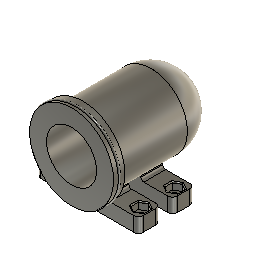
POP_MainBody_Extended_Feet (Autodesk Fusion 360 design; units mm, degrees)
Autodesk Fusion 360 part; units mm, degrees
sketch "Sketch1" plane through (0, 0, 0) normal (0, 1, 0) x (1, 0, 0)
  circle A0 centre (0, 0) radius 22
  circle A1 centre (0, 0) radius 32
  dimension "d1" = 44
  dimension "d2" = 10
  constraint coincident A0.centre A1.centre
  measures "d1" diameter of A0
extrude "Extrude1" add sketch "Sketch1" along normal blind 70 makes body 1
sketch "Sketch2" plane through (0, 0, 0) normal (0, 0, 1) x (1, 0, 0)
  line L0 (0, 0) -> (0, 97.6409) construction
  line L1 (0, 69.4626) -> (31, 69.4626)
  arc A0 (0, 91.4626) -> (-22, 69.4626) centre (0, 69.4626) ccw
  arc A1 (0, 101.4626) -> (-32, 69.4626) centre (0, 69.4626) ccw
  line L2 (0, 69.4626) -> (-32, 69.4626) construction
  line L3 (31, 69.4626) -> (21, 69.4626)
  line L4 (-22, 69.4626) -> (-32, 69.4626)
  line L5 (0, 91.4626) -> (0, 101.4626)
  dimension "d7" = 32
  dimension "d8" = 22
  constraint coincident L0.start origin
  constraint vertical L0
  constraint coincident L1.start L0
  constraint coincident L1.start A0.centre
  constraint perpendicular L0 L1
  constraint concentric A0 A1
  constraint coincident L1 L3.end
  constraint perpendicular L0 L2
  constraint coincident L2 A0.end
  measures "d7" radius of A1
  measures "d8" radius of A0
revolve "Revolve1" add sketch "Sketch2" angle 360 about axis through (0, 0, 0) along (0, 1, 0) bodies 1
sketch "Sketch3" plane through (0, 0, 0) normal (0, -1, 0) x (1, 0, 0)
  circle A0 centre (0, 0) radius 22
  circle A1 centre (0, 0) radius 32
  circle A2 centre (0, 0) radius 25.146 construction
  circle A3 centre (0, 0) radius 28.702 construction
  dimension "d10" = 50.292
  dimension "d11" = 57.404
  constraint coincident A0.centre A1.centre
  measures "d10" diameter of A2
  measures "d11" diameter of A3
ref_plane "WorkPlane1" through (0, 37.5401, -32) normal (0, 0, -1) x (1, 0, 0)
sketch "Sketch4" plane through (0, 37.5401, -32) normal (0, 0, -1) x (1, 0, 0)
  line L0 (45, 23.5401) -> (-45, 23.5401)
  line L1 (-45, 23.5401) -> (-45, 4.2401)
  line L2 (-45, 4.2401) -> (45, 4.2401)
  line L3 (45, 4.2401) -> (45, 23.5401)
  line L4 (45, 23.5401) -> (-45, 4.2401) construction
  line L5 (-45, 23.5401) -> (45, 4.2401) construction
  line L6 (0, 0) -> (0, 37.5401) construction
  line L7 (0, 0) -> (0, -48.773) construction
  circle A0 centre (-37.35, 13.8901) radius 3.302
  circle A1 centre (37.35, 13.8901) radius 3.302
  point P0 (0, 13.8901)
  point P1 (0, 37.5401)
  dimension "d13" = 90
  dimension "d14" = 19.3
  dimension "d15" = 14
  dimension "d16" = 6.604
  dimension "d17" = 7.65
  dimension "d18" = 6.604
  dimension "d19" = 7.65
  dimension "d20" = 9.65
  dimension "d21" = 9.65
  constraint horizontal L0
  constraint perpendicular L0 L1
  constraint parallel L0 L2
  constraint parallel L1 L3
  constraint coincident L4 P0
  constraint coincident L5 P0
  constraint midpoint L5 P0
  constraint coincident L6.start L7.start
  constraint perpendicular L0 L6
  constraint coincident P0 L6
  constraint parallel L6 L7
  constraint coincident P1 L6.end
  measures "d13" distance of L0.start L0.end
  measures "d14" distance of L0.end L1.end
  measures "d15" distance of L0 P1
  measures "d16" diameter of A0
  measures "d17" distance of L1 A0.centre
  measures "d18" diameter of A1
  measures "d19" distance of L3 A1.centre
  measures "d20" distance of L0 A0.centre
  measures "d21" distance of L0 A1.centre
extrude "Extrude2" add sketch "Sketch4" against normal blind 12.7 from surface at 12.7 separate body makes body 2
sketch "Sketch11" plane through (0, 0, -32) normal (0, 0, 1) x (-1, 0, 0)
  circle A0 centre (-37.35, -23.65) radius 3.302
  circle A1 centre (37.35, -23.65) radius 3.302
  line L0 (-45, -14) -> (-45, -33.3)
  line L1 (-45, -33.3) -> (45, -33.3)
  line L2 (45, -33.3) -> (45, -14)
  line L3 (45, -14) -> (-45, -14)
  line L4 (-42.938, -20.4238) -> (-42.938, -26.8762)
  line L5 (-42.938, -26.8762) -> (-37.35, -30.1025)
  line L6 (-37.35, -30.1025) -> (-31.762, -26.8762)
  line L7 (-31.762, -26.8762) -> (-31.762, -20.4238)
  line L8 (-31.762, -20.4238) -> (-37.35, -17.1975)
  line L9 (-37.35, -17.1975) -> (-42.938, -20.4238)
  line L10 (0, -33.3) -> (0, -14) construction
  line L11 (42.938, -26.8762) -> (37.35, -30.1025)
  line L12 (42.938, -20.4238) -> (42.938, -26.8762)
  line L13 (37.35, -17.1975) -> (42.938, -20.4238)
  line L14 (31.762, -20.4238) -> (37.35, -17.1975)
  line L15 (31.762, -26.8762) -> (31.762, -20.4238)
  line L16 (37.35, -30.1025) -> (31.762, -26.8762)
  point P0 (-37.35, -23.65)
  dimension "d77" = 11.176
  constraint coincident P0 A0.centre
  constraint vertical L4
  constraint midpoint L1 L10.start
  constraint midpoint L3 L10.end
  constraint symmetric L4.start L10 L12.start
  constraint symmetric L4.end L10 L11.start
  constraint symmetric L5.end L10 L11.end
  constraint symmetric L6.end L10 L15.start
  constraint symmetric L7.end L10 L14.start
  constraint symmetric L8.end L10 L13.start
  measures "d77" distance of L4 L7
extrude "Extrude9" cut sketch "Sketch11" against normal blind 6.35 contours L4 L5 L6 L7 L8 L9 | L11 L12 L13 L14 L15 L16 bodies 2
fillet "Fillet2" radius 4 4 edges at (-45, 14, -38.35) (-45, 33.3, -38.35) (45, 14, -38.35) (45, 33.3, -38.35) on bodies 2
sketch "Sketch12" plane through (0, 0, -32) normal (0, 0, 1) x (-1, 0, 0)
  arc A0 (-45, -29.3) -> (-41, -33.3) centre (-41, -29.3) ccw
  line L0 (-41, -33.3) -> (41, -33.3)
  arc A1 (41, -33.3) -> (45, -29.3) centre (41, -29.3) ccw
  line L1 (45, -29.3) -> (45, -18)
  arc A2 (45, -18) -> (41, -14) centre (41, -18) ccw
  line L2 (41, -14) -> (-41, -14)
  arc A3 (-41, -14) -> (-45, -18) centre (-41, -18) ccw
  line L3 (-45, -18) -> (-45, -29.3)
  line L4 (-42.938, -26.8762) -> (-42.938, -20.4238)
  line L5 (-42.938, -20.4238) -> (-37.35, -17.1975)
  line L6 (-37.35, -17.1975) -> (-31.762, -20.4238)
  line L7 (-31.762, -20.4238) -> (-31.762, -26.8762)
  line L8 (-31.762, -26.8762) -> (-37.35, -30.1025)
  line L9 (-37.35, -30.1025) -> (-42.938, -26.8762)
  line L10 (42.938, -20.4238) -> (42.938, -26.8762)
  line L11 (42.938, -26.8762) -> (37.35, -30.1025)
  line L12 (37.35, -30.1025) -> (31.762, -26.8762)
  line L13 (31.762, -26.8762) -> (31.762, -20.4238)
  line L14 (31.762, -20.4238) -> (37.35, -17.1975)
  line L15 (37.35, -17.1975) -> (42.938, -20.4238)
  line L16 (0, -14) -> (0, -33.3) construction
  line L17 (-17.145, -14) -> (17.145, -14)
  line L18 (17.145, -14) -> (17.145, -33.3)
  line L19 (17.145, -33.3) -> (-17.145, -33.3)
  line L20 (-17.145, -33.3) -> (-17.145, -14)
  line L21 (-17.145, -14) -> (17.145, -33.3) construction
  line L22 (17.145, -14) -> (-17.145, -33.3) construction
  point P0 (0, -23.65)
  dimension "d80" = 34.29
  constraint midpoint L2 L16.start
  constraint midpoint L0 L16.end
  constraint horizontal L17
  constraint perpendicular L17 L18
  constraint parallel L17 L19
  constraint parallel L18 L20
  constraint coincident L21 P0
  constraint coincident L22 P0
  constraint coincident L2 L17.start
  constraint midpoint L16 P0
  measures "d80" distance of L18.end L19.end
extrude "Extrude10" add sketch "Sketch12" along normal blind 5.08 contours L0 L2 L17 L18 L19 L20 bodies 1 2
fillet "Fillet8" radius 2.54 2 edges at (17.145, 23.65, -27.0194) (-17.145, 23.65, -27.0194) on bodies 1
fillet "Fillet9" radius 2.54 2 edges at (-17.145, 23.65, -32) (17.145, 23.65, -32) on bodies 1
fillet "Fillet10" chord length 1.27 12 edges at (31.762, 23.65, -32) (34.556, 28.4893, -32) (34.556, 18.8107, -32) (40.144, 18.8107, -32) (42.938, 23.65, -32) (40.144, 28.4893, -32) (-34.556, 28.4893, -32) (-31.762, 23.65, -32) (-34.556, 18.8107, -32) (-40.144, 18.8107, -32) (-42.938, 23.65, -32) (-40.144, 28.4893, -32) on bodies 1
sketch "Sketch5" plane through (0, 0, 0) normal (0, -1, 0) x (1, 0, 0)
  circle A0 centre (0, 0) radius 37
  circle A1 centre (0, 0) radius 30.8058
  dimension "d31" = 74
  constraint coincident A0.centre A1.centre
  constraint concentric A0 A1
  measures "d31" diameter of A0
extrude "Extrude3" add sketch "Sketch5" against normal blind 10 bodies 1
coil "CoilPrimitive1" add diameter 74 section circle size 2 on centre turns 1.5 pitch 6.66667 right hand placed x (1, 0, 0) y (0, 0, -1) z (0, 1, 0) at (0, 0, 0) separate body makes body 3
move_body "Move1" bodies 3 to x (1, 0, 0) y (0, 1, 0) z (0, 0, 1) at (0, -1.5, 0)
combine "Combine1" operation add target body 1 tool bodies 3
sketch "Sketch7" plane through (0, 0, 0) normal (0, -1, 0) x (1, 0, 0)
  circle A0 centre (0, 0) radius 22
  circle A1 centre (0, 0) radius 50.9902
  spline S0 degree 3 poles (-26.163, -26.163) (-26.1604, -26.1604) (-26.1574, -26.1584) (-26.1496, -26.1548) (-26.1447, -26.1537) (-26.1307, -26.1522) (-26.1207, -26.1533) (-26.0884, -26.1593) (-26.0612, -26.1697) (-25.9436, -26.2231) (-25.8159, -26.3056) (-24.8505, -26.9737) (-23.1166, -28.4335) (-15.2241, -33.4022) (-10.4173, -34.7745) (-2.6703, -36.1642) (1.5215, -36.2078) (5.6316, -35.5568) knots 3.244354 3.244354 3.244354 3.244354 3.253489 3.253489 3.265817 3.265817 3.288767 3.288767 3.348492 3.348492 3.563904 3.563904 4.976735 4.976735 7.989432 7.989432 11.394709 11.394709 11.394709 11.394709
  spline S1 degree 3 poles (5.6316, -35.5568) (6.3802, -35.4382) (7.1261, -35.2966) (12.4413, -34.1173) (16.7708, -32.2508) (24.9958, -26.7102) (27.9306, -23.4279) (30.9522, -19.5432) (31.772, -18.3009) (32.5635, -17.1873) (32.7513, -16.9397) (32.8911, -16.8205) (32.9135, -16.8052) (32.9389, -16.796) (32.9458, -16.7943) (32.9569, -16.7943) (32.9612, -16.795) (32.9659, -16.797) (32.9666, -16.7973) (32.9672, -16.7976) knots 11.394709 11.394709 11.394709 11.394709 12.01493 12.01493 15.836449 15.836449 20.097613 20.097613 22.736598 22.736598 23.856469 23.856469 24.088678 24.088678 24.16644 24.16644 24.216158 24.216158 24.224748 24.224748 24.224748 24.224748
  arc A2 (32.9672, -16.7976) -> (-26.163, -26.163) centre (0, 0) ccw
  constraint concentric A0 A1
extrude "Extrude4" cut sketch "Sketch7" along normal blind 15 contours A1 | S0 S1 A2 bodies 1
pattern_linear "R-Pattern1" count 2 spacing 30 along (0, 1, 0) of "Extrude2", "Extrude9", "Fillet2", "Extrude10", "Fillet8", "Fillet9", "Fillet10"
